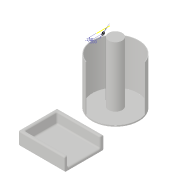
# Autodesk Inventor part: Nicole's Ideas
Saved by Autodesk Inventor 2018 (Build 220112000, 112)
## iProperties
Created: 2019-10-09
Part Number: Nicole's Ideas
Material: Generic
Document SubType Name: Modeling
Designer: ball
Density: 1 g/cm^3
Appearance: Default
Author: ball
Autodesk Inventor part; units mm, degrees
ref_plane "YZ Plane" through (0, 0, 0) normal (1, 0, 0) x (0, 1, 0)
ref_plane "XZ Plane" through (0, 0, 0) normal (0, 1, 0) x (-1, 0, 0)
ref_plane "XY Plane" through (0, 0, 0) normal (0, 0, 1) x (1, 0, 0)
sketch "Sketch1" plane through (0, 0, 0) normal (0, 1, 0) x (-1, 0, 0)
  line L0 (0, 0) -> (-88.265, 0)
  line L1 (-88.265, 0) -> (-88.265, 73.8124)
  line L2 (-88.265, 73.8124) -> (0, 73.8124)
  line L3 (0, 73.8124) -> (0, 0)
  dimension "d0" = 88.265
  dimension "d1" = 73.8124
  constraints: 8 end point, 2 parallel, 1 horizontal, 1 perpendicular
  measures "d0" distance of L1.end L2.end
  measures "d1" distance of L0.end L1.end
extrude "Extrusion1" add sketch "Sketch1" along normal blind 25.0444
sketch "Sketch2" plane through (0, 25.0444, 0) normal (0, 1, 0) x (1, 0, 0)
  line L0 (88.265, -6.35) -> (6.35, -6.35)
  line L1 (6.35, -6.35) -> (6.35, -67.4624)
  line L2 (6.35, -67.4624) -> (88.265, -67.4624)
  line L3 (88.265, -67.4624) -> (88.265, -6.35)
  line L4 (88.265, -73.8124) -> (88.265, 0) projected
  line L5 (0, 0) -> (0, -73.8124) projected
  line L6 (88.265, 0) -> (0, 0) projected
  line L7 (0, -73.8124) -> (88.265, -73.8124) projected
  dimension "d4" = 0
  dimension "d5" = 6.35
  dimension "d6" = 6.35
  dimension "d7" = 6.35
  constraints: 8 end point, 2 parallel, 1 horizontal, 1 perpendicular
  measures "d4" distance between parallel lines of L3 L4
  measures "d5" distance between parallel lines of L5 L1
  measures "d6" distance between parallel lines of L6 L0
  measures "d7" distance between parallel lines of L7 L2
extrude "Extrusion2" cut sketch "Sketch2" against normal blind 19.9644 contours L3 L2 L1 L0
fillet "Fillet1" radius 2.54 18 edges at (47.3075, 5.08, 67.4624) (6.35, 5.08, 36.9062) (47.3075, 5.08, 6.35) (0, 0, 36.9062) (0, 25.0444, 36.9062) (44.1325, 0, 0) (44.1325, 25.0444, 0) (47.3075, 25.0444, 67.4624) (44.1325, 25.0444, 73.8124) (6.35, 25.0444, 36.9062) (88.265, 25.0444, 70.6374) (88.265, 25.0444, 3.175) (47.3075, 25.0444, 6.35) (44.1325, 0, 73.8124) (6.35, 15.0622, 6.35) (6.35, 15.0622, 67.4624) (0, 12.5222, 0) (0, 12.5222, 73.8124)
fillet "Fillet2" radius 2.54 7 edges at (88.265, 5.8239, 7.0939) (88.265, 5.08, 36.9062) (88.265, 5.8239, 66.7185) (88.265, 15.0622, 67.4624) (87.5211, 24.3005, 68.2063) (87.5211, 24.3005, 5.6061) (88.265, 15.0622, 6.35)
sketch "Sketch3" plane through (0, 0, 0) normal (0, -1, 0) x (1, 0, 0)
  circle A0 centre (30.1625, -80.9625) radius 44.45
  point P0 (0, 0)
  dimension "d12" = 88.9
  constraints: 1 centre point
  measures "d12" diameter of A0
extrude "Extrusion3" add sketch "Sketch3" against normal blind 88.9
sketch "Sketch4" plane through (30.1625, 88.9, -80.9625) normal (0, 1, 0) x (1, 0, 0)
  circle A0 centre (0, 0) radius 43.18
  point P0 (-30.1625, -80.9625)
  dimension "d15" = 86.36
  constraints: 1 centre point
  measures "d15" diameter of A0
extrude "Extrusion4" cut sketch "Sketch4" against normal blind 86.36
sketch "Sketch5" plane through (30.1625, 88.9, -80.9625) normal (0, 1, 0) x (1, 0, 0)
  line L0 (44.45, 0) -> (44.45, -44.45)
  line L1 (44.45, -44.45) -> (0, -44.45)
  line L2 (44.45, -44.45) -> (-14.2875, -44.45)
  line L3 (-14.2875, -44.45) -> (-14.2875, 14.2875)
  line L4 (-14.2875, 14.2875) -> (44.45, 14.2875)
  line L5 (44.45, 14.2875) -> (44.45, -44.45)
  point P0 (-30.1625, -80.9625)
  constraints: 12 end point, 2 parallel, 1 horizontal, 1 perpendicular
extrude "Extrusion5" cut sketch "Sketch5" against normal blind 86.36
sketch "Sketch6" plane through (30.1625, 2.54, -80.9625) normal (0, 1, 0) x (1, 0, 0)
  circle A0 centre (0, 0) radius 12.954
  point P0 (-30.1625, -80.9625)
  dimension "d20" = 25.908
  constraints: 1 centre point
  measures "d20" diameter of A0
extrude "Extrusion6" add sketch "Sketch6" along normal blind 114.3
sketch "Sketch7" plane through (6.35, 7.62, 64.9224) normal (1, 0, 0) x (0, 0, -1)
  circle A0 centre (146.05, 102.87) radius 2.54
  line L0 (158.8389, 109.22) -> (132.9309, 109.22) projected
  point P0 (64.9224, -7.62)
  dimension "d23" = 5.08
  dimension "d24" = 6.35
  constraints: 1 centre point
  measures "d23" diameter of A0
  measures "d24" distance from line of L0 A0.centre
body "Solid1"
